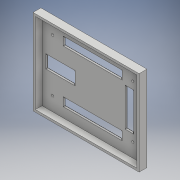
# Autodesk Inventor part: Platform-bottom
Saved by Autodesk Inventor 2017 (Build 210142000, 142)
## iProperties
Created: 2018-03-19
Part Number: Platform-bottom
Material: Generic
Document SubType Name: Modeling
Designer: Arjuna
Density: 1 g/cm^3
Appearance: Default
Author: Arjuna
## iProperties of the stored document Platform-bottom_3DPrint.ipt
Created: 2018-03-30
Part Number: Platform-bottom_3DPrint
Material: Generic
Document SubType Name: Modeling
Designer: Arjuna
Density: 1 g/cm^3
Appearance: Default
Author: Arjuna
Autodesk Inventor part; units mm, degrees
ref_plane "YZ Plane" through (0, 0, 0) normal (1, 0, 0) x (0, 1, 0)
ref_plane "XZ Plane" through (0, 0, 0) normal (0, 1, 0) x (-1, 0, 0)
ref_plane "XY Plane" through (0, 0, 0) normal (0, 0, 1) x (1, 0, 0)
sketch "Sketch1" plane through (0, 0, 0) normal (0, 1, 0) x (-1, 0, 0)
  line L0 (115, 92.5) -> (-115, 92.5)
  line L1 (-115, 92.5) -> (-115, -92.5)
  line L2 (-115, -92.5) -> (115, -92.5)
  line L3 (115, -92.5) -> (115, 92.5)
  point P0 (0, 0)
  dimension "d0" = 185
  dimension "d1" = 230
  dimension "d2" = 92.5
  dimension "d3" = 115
  constraints: 8 end point, 2 parallel, 1 horizontal, 1 perpendicular
  measures "d0" distance of L2.end L0.start
  measures "d1" distance of L1.end L2.end
  measures "d2" distance from line of point (0, 0) L0
  measures "d3" distance from line of point (0, 0) L3
extrude "Extrusion1" add sketch "Sketch1" along normal blind 17
sketch "Sketch2" plane through (0, 0, 0) normal (0, -1, 0) x (1, 0, 0)
  line L0 (-115, 92.5) -> (115, 92.5) projected
  line L1 (-115, -92.5) -> (-115, 92.5) projected
  line L2 (115, -92.5) -> (-115, -92.5) projected
  line L3 (115, 92.5) -> (115, -92.5) projected
  line L4 (-110, -87.5) -> (110, -87.5)
  line L5 (110, -87.5) -> (110, 87.5)
  line L6 (110, 87.5) -> (-110, 87.5)
  line L7 (-110, 87.5) -> (-110, -87.5)
  point P0 (0, 0)
  dimension "d6" = 5
  dimension "d7" = 5
  dimension "d8" = 5
  dimension "d9" = 5
  constraints: 8 end point, 2 parallel, 1 horizontal, 1 perpendicular
  measures "d6" distance between parallel lines of L4 L2
  measures "d7" distance between parallel lines of L7 L1
  measures "d8" distance between parallel lines of L0 L6
  measures "d9" distance between parallel lines of L3 L5
extrude "Extrusion2" cut sketch "Sketch2" against normal blind 14.5 contours L7 L6 L5 L4
sketch "Sketch3" plane through (0, 17, 0) normal (0, 1, 0) x (1, 0, 0)
  line L0 (-100, -12.5) -> (-40, -12.5)
  line L1 (-40, -12.5) -> (-40, 12.5)
  line L2 (-40, 12.5) -> (-100, 12.5)
  line L3 (-100, 12.5) -> (-100, -12.5)
  point P0 (0, 0)
  dimension "d12" = 40
  dimension "d13" = 60
  dimension "d14" = 12.5
  dimension "d15" = 25
  constraints: 8 end point, 2 parallel, 1 horizontal, 1 perpendicular
  measures "d12" distance from line of L1 point (0, 0)
  measures "d13" distance of L1.end L2.end
  measures "d14" distance from line of point (0, 0) L0
  measures "d15" distance of L2.end L0.start
extrude "Extrusion3" cut sketch "Sketch3" against normal through all
sketch "Sketch4" plane through (0, 17, 0) normal (0, 1, 0) x (1, 0, 0)
  line L0 (-87, -64.5) -> (87, -64.5)
  line L1 (87, -64.5) -> (87, 64.5)
  line L2 (87, 64.5) -> (-87, 64.5)
  line L3 (-87, 64.5) -> (-87, -64.5)
  line L4 (-72, -49.5) -> (72, -49.5)
  line L5 (72, -49.5) -> (72, 49.5)
  line L6 (72, 49.5) -> (-72, 49.5)
  line L7 (-72, 49.5) -> (-72, -49.5)
  line L8 (-87, -39.5) -> (-72, -39.5)
  line L9 (-87, 39.5) -> (-72, 39.5)
  line L10 (-62, 49.5) -> (-62, 64.5)
  line L11 (-62, -49.5) -> (-62, -64.5)
  line L12 (62, -49.5) -> (62, -64.5)
  line L13 (72, -39.5) -> (87, -39.5)
  line L14 (72, 39.5) -> (87, 39.5)
  line L15 (62, 49.5) -> (62, 64.5)
  point P0 (0, 0)
  dimension "d18" = 129
  dimension "d19" = 174
  dimension "d20" = 64.5
  dimension "d21" = 87
  dimension "d22" = 15
  dimension "d23" = 15
  dimension "d24" = 15
  dimension "d25" = 15
  dimension "d26" = 25
  dimension "d27" = 25
  dimension "d28" = 25
  dimension "d29" = 25
  dimension "d30" = 25
  dimension "d31" = 25
  dimension "d32" = 25
  dimension "d33" = 25
  constraints: 32 end point, 16 point on line, 10 perpendicular, 4 parallel, 2 horizontal
  measures "d18" distance of L2.end L0.start
  measures "d19" distance of L0.start L0.end
  measures "d20" distance from line of point (0, 0) L0
  measures "d21" distance from line of point (0, 0) L1
  measures "d22" distance between parallel lines of L7 L3
  measures "d23" distance between parallel lines of L4 L0
  measures "d24" distance between parallel lines of L2 L6
  measures "d25" distance between parallel lines of L1 L5
  measures "d26" distance between parallel lines of L0 L8
  measures "d27" distance between parallel lines of L3 L11
  measures "d28" distance between parallel lines of L2 L9
  measures "d29" distance between parallel lines of L3 L10
  measures "d30" distance between parallel lines of L1 L12
  measures "d31" distance between parallel lines of L13 L0
  measures "d32" distance between parallel lines of L2 L14
  measures "d33" distance between parallel lines of L1 L15
extrude "Extrusion4" cut sketch "Sketch4" against normal through all contours L11 L4 L12 L0 | L13 L5 L14 L1 | L2 L15 L6 L10
sketch "Sketch5" plane through (0, 17, 0) normal (0, 1, 0) x (1, 0, 0)
  circle A0 centre (-87, -57) radius 2.5
  circle A1 centre (-87, 57) radius 2.5
  circle A2 centre (87, -57) radius 2.5
  circle A3 centre (87, 57) radius 2.5
  point P0 (0, 0)
  dimension "d36" = 5
  dimension "d37" = 57
  dimension "d38" = 87
  dimension "d39" = 5
  dimension "d40" = 87
  dimension "d41" = 57
  dimension "d42" = 5
  dimension "d43" = 57
  dimension "d44" = 87
  dimension "d45" = 5
  dimension "d46" = 57
  dimension "d47" = 87
  constraints: 4 centre point
  measures "d36" diameter of A0
  measures "d37" vertical distance of point (0, 0) A0.centre
  measures "d38" horizontal distance of A0.centre point (0, 0)
  measures "d39" diameter of A1
  measures "d40" horizontal distance of point (0, 0) A1.centre
  measures "d41" vertical distance of A1.centre point (0, 0)
  measures "d42" diameter of A2
  measures "d43" vertical distance of point (0, 0) A2.centre
  measures "d44" horizontal distance of point (0, 0) A2.centre
  measures "d45" diameter of A3
  measures "d46" vertical distance of point (0, 0) A3.centre
  measures "d47" horizontal distance of point (0, 0) A3.centre
extrude "Extrusion5" cut sketch "Sketch5" against normal through all
fillet "Fillet1" radius 2 16 edges at (72, 14.5, 0) (87, 14.5, 0) (79.5, 14.5, 39.5) (79.5, 14.5, -39.5) (0, 14.5, -49.5) (0, 14.5, -64.5) (62, 14.5, -57) (-62, 14.5, -57) (-70, 14.5, -12.5) (-70, 14.5, 12.5) (-100, 14.5, 0) (-40, 14.5, 0) (0, 14.5, 49.5) (-62, 14.5, 57) (0, 14.5, 64.5) (62, 14.5, 57)
fillet "Fillet2" radius 1 32 edges at (-62, 16.75, 64.5) (-62.5858, 15.0858, 65.0858) (-62, 16.75, 49.5) (-62.5858, 15.0858, 48.9142) (62, 16.75, 64.5) (62.5858, 15.0858, 65.0858) (62, 16.75, 49.5) (62.5858, 15.0858, 48.9142) (72, 16.75, 39.5) (71.4142, 15.0858, 40.0858) (87, 16.75, 39.5) (87.5858, 15.0858, 40.0858) (72, 16.75, -39.5) (71.4142, 15.0858, -40.0858) (87, 16.75, -39.5) (87.5858, 15.0858, -40.0858) (62, 16.75, -49.5) (62.5858, 15.0858, -48.9142) (62, 16.75, -64.5) (62.5858, 15.0858, -65.0858) (-62, 16.75, -64.5) (-62.5858, 15.0858, -65.0858) (-62, 16.75, -49.5) (-62.5858, 15.0858, -48.9142) (-40, 16.75, -12.5) (-39.4142, 15.0858, -13.0858) (-40, 16.75, 12.5) (-39.4142, 15.0858, 13.0858) (-100, 16.75, 12.5) (-100.5858, 15.0858, 13.0858) (-100, 16.75, -12.5) (-100.5858, 15.0858, -13.0858)
equation "\"d2\" = 0.5 * d0"
equation "\"d3\" = 0.5 * d1"
equation "\"d7\" = d6"
equation "\"d8\" = d6"
equation "\"d9\" = d6"
equation "\"d14\" = 0.5 * d15"
equation "\"d20\" = 0.5 * d18"
equation "\"d21\" = 0.5 * d19"
equation "\"d23\" = d22"
equation "\"d24\" = d22"
equation "\"d25\" = d22"
equation "\"d27\" = d26"
equation "\"d28\" = d26"
equation "\"d29\" = d26"
equation "\"d30\" = d26"
equation "\"d31\" = d26"
equation "\"d32\" = d26"
equation "\"d33\" = d26"
equation "\"d39\" = d36"
equation "\"d40\" = d38"
equation "\"d41\" = d37"
equation "\"d42\" = d36"
equation "\"d43\" = d37"
equation "\"d44\" = d38"
equation "\"d45\" = d36"
equation "\"d46\" = d37"
equation "\"d47\" = d38"
body "Solid1"
